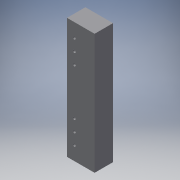
# Autodesk Inventor part: RodBase
Saved by Autodesk Inventor 2017 SP1 (Build 210196100, 196)
## iProperties
Created: 2017-10-17
Part Number: RodBase
Material: Generic
Document SubType Name: Modeling
Designer: 1452927
Density: 1 g/cm^3
Appearance: Default
Author: 1452927
Autodesk Inventor part; units mm, degrees
ref_plane "YZ Plane" through (0, 0, 0) normal (1, 0, 0) x (0, 1, 0)
ref_plane "XZ Plane" through (0, 0, 0) normal (0, 1, 0) x (-1, 0, 0)
ref_plane "XY Plane" through (0, 0, 0) normal (0, 0, 1) x (1, 0, 0)
sketch "Sketch1" plane through (0, 0, 0) normal (0, 1, 0) x (-1, 0, 0)
  line L0 (19.05, -83) -> (19.05, 83)
  line L1 (-19.05, 83) -> (-19.05, -83)
  circle A0 centre (0, 0) radius 11.5094
  line L2 (0, 0) -> (-0.4877, 3.251) construction
  line L3 (0, 0) -> (0, 63.5) construction
  line L4 (0, 0) -> (0, -63.5) construction
  circle A1 centre (0, 63.5) radius 3.5719
  circle A2 centre (0, -63.5) radius 3.5719
  line L5 (19.05, 83) -> (-19.05, 83)
  line L6 (19.05, -83) -> (-19.05, -83)
  dimension "d2" = 23.0188
  dimension "d4" = 63.5
  dimension "d5" = 63.5
  dimension "d6" = 7.1437
  dimension "d7" = 7.1437
  constraints: 14 end point, 3 centre point, 3 coincident, 2 perpendicular, 2 vertical, 1 parallel
  measures "d2" diameter of A0
  measures "d4" distance of L2.start L3.end
  measures "d5" distance of L2.start L4.end
  measures "d6" diameter of A1
  measures "d7" diameter of A2
extrude "Extrusion1" add sketch "Sketch1" along normal blind 25.4
sketch "Sketch6" plane through (0, 0, 0) normal (0, -1, 0) x (1, 0, 0)
  circle A0 centre (0, 63.5) radius 3.5719 projected
  circle A1 centre (0, 63.5) radius 3.5719
  circle A2 centre (0, -63.5) radius 3.5719 projected
  circle A3 centre (0, -63.5) radius 3.5719
  circle A4 centre (0, 0) radius 11.5094
  constraints: 3 centre point, 3 coincident
extrude "Extrusion8" add sketch "Sketch6" against normal blind 5
sketch "Sketch8" plane through (0, 25.4, 0) normal (0, 1, 0) x (1, 0, 0)
  point P0 (0, 0)
sketch "Sketch9" plane through (0, 25.4, 0) normal (0, 1, 0) x (1, 0, 0)
  circle A0 centre (0, 0) radius 11.5094 projected
  line L0 (-19.05, 83) -> (-19.05, -83) projected
  line L1 (19.05, -83) -> (19.05, 83) projected
  circle A1 centre (0, -63.5) radius 3.5719 projected
sketch "Sketch12" plane through (0, 25.4, 0) normal (0, 1, 0) x (1, 0, 0)
  point P0 (0, 0)
sketch "Sketch13" plane through (0, 25.4, 0) normal (0, 1, 0) x (1, 0, 0)
  circle A0 centre (-9.05, -64) radius 1.905
  circle A1 centre (-9.05, -48) radius 1.905
  circle A2 centre (-9.05, -32) radius 1.905
  circle A3 centre (-9.05, 32) radius 1.905
  circle A4 centre (-9.05, 48) radius 1.905
  circle A5 centre (-9.05, 64) radius 1.905
  point P0 (0, 0)
  dimension "d67" = 3.81
  dimension "d68" = 3.81
  dimension "d69" = 3.81
  dimension "d70" = 3.81
  dimension "d71" = 3.81
  dimension "d72" = 3.81
  constraints: 6 centre point, 6 other
  measures "d67" diameter of A0
  measures "d68" diameter of A1
  measures "d69" diameter of A2
  measures "d70" diameter of A3
  measures "d71" diameter of A4
  measures "d72" diameter of A5
extrude "Extrusion14" cut sketch "Sketch13" against normal up to next
sketch "Sketch14" plane through (19.05, 0, -83) normal (0, 0, -1) x (-1, 0, 0)
  line L0 (0, 0) -> (0, 25.4) projected
  line L1 (38.1, 0) -> (38.1, 25.4) projected
  line L2 (0, 25.4) -> (38.1, 25.4)
  line L3 (38.1, 25.4) -> (38.1, 16.2292)
  line L4 (38.1, 16.2292) -> (0, 16.2292)
  line L5 (0, 16.2292) -> (0, 25.4)
  point P0 (19.05, 0)
  constraints: 8 end point, 2 parallel, 1 horizontal, 1 perpendicular, 1 point on line
extrude "Extrusion15" cut sketch "Sketch14" against normal up to next
body "Solid1"
